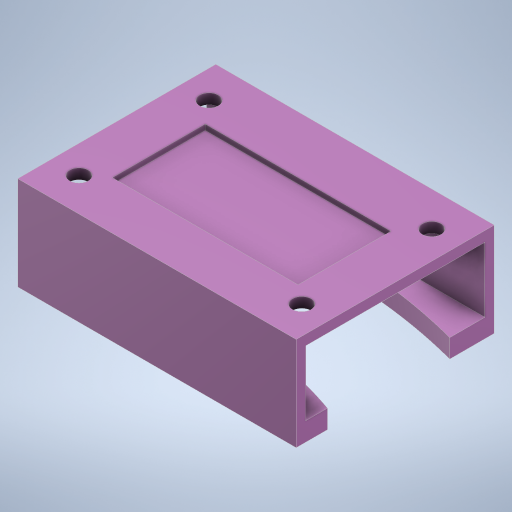
# Autodesk Inventor part: Battery Cage
Saved by Autodesk Inventor 2023 (Build 270158000, 158)
## iProperties
Created: 2022-10-27
Part Number: Battery Cage
Material: PLA Plastic
Document SubType Name: Modeling
Designer: cheng
Density: 1.25002 g/cm^3
Appearance: Generic
Mass: 171.099 g
Surface Area: 610.398 cm^2
Volume: 136.877 cm^3
Author: cheng
Autodesk Inventor part; units mm, degrees
ref_plane "YZ Plane" through (0, 0, 0) normal (1, 0, 0) x (0, 1, 0)
ref_plane "XZ Plane" through (0, 0, 0) normal (0, 1, 0) x (-1, 0, 0)
ref_plane "XY Plane" through (0, 0, 0) normal (0, 0, 1) x (1, 0, 0)
sketch "Sketch1" plane through (0, 0, 0) normal (0, 1, 0) x (-1, 0, 0)
  line L0 (75, -60) -> (-75, -60)
  line L1 (-75, -60) -> (-75, 60)
  line L2 (-75, 60) -> (75, 60)
  line L3 (75, 60) -> (75, -60)
  line L4 (75, -60) -> (-75, 60) construction
  line L5 (-75, -60) -> (75, 60) construction
  point P0 (0, 0)
  dimension "d0" = 120
  dimension "d1" = 150
  constraints: 12 end point, 2 midpoint, 2 parallel, 1 horizontal, 1 perpendicular
  measures "d0" distance of L2.end L0.start
  measures "d1" distance of L0.start L0.end
extrude "Extrusion1" add sketch "Sketch1" along normal blind 50.5
sketch "Sketch14" plane through (0, 0, 0) normal (0, 1, 0) x (1, 0, 0)
  line L0 (-75, -60) -> (75, -60) projected
  line L1 (75, -60) -> (75, 60) projected
  line L2 (75, 60) -> (-75, 60) projected
  line L3 (-75, 60) -> (-75, -60) projected
  line L4 (0, 0) -> (0, -250) construction
  circle A0 centre (0, -250) radius 260
  circle A1 centre (0, -250) radius 291.5
  circle A2 centre (0, -250) radius 228.5
  point P0 (75, 31.6864)
  point P1 (-75, 31.6864)
  point P2 (-75, -34.1592)
  point P3 (75, -34.1592)
  dimension "d52" = 250
  dimension "d53" = 520
  dimension "d54" = 583
  dimension "d55" = 457
  constraints: 4 coincident, 3 centre point, 2 end point, 1 vertical
  measures "d52" distance of L4.start L4.end
  measures "d53" diameter of A0
  measures "d54" diameter of A1
  measures "d55" diameter of A2
extrude "Extrusion13" cut sketch "Sketch14" along normal blind 45 contours L3 A0 L1 A2 | L3 A1 L1 A0 picked at (-61.8874, -8.4536) picked at (67.9829, 11.6585)
sketch "Sketch15" plane through (0, 45, 0) normal (0, -1, 0) x (1, 0, 0)
  line L0 (0, 0) -> (0, 250) construction
  circle A0 centre (0, 250) radius 260
  circle A1 centre (0, 250) radius 302.5
  circle A2 centre (0, 250) radius 217.5
  line L1 (-75, 60) -> (75, 60) projected
  line L2 (75, 60) -> (75, -60) projected
  line L3 (75, -60) -> (-75, -60) projected
  line L4 (-75, -60) -> (-75, 60) projected
  point P0 (-75, -43.055)
  point P1 (75, -43.055)
  point P2 (75, 45.8401)
  point P3 (-75, 45.8401)
  dimension "d58" = 250
  dimension "d59" = 520
  dimension "d60" = 605
  dimension "d61" = 435
  constraints: 4 coincident, 3 centre point, 2 end point, 1 vertical
  measures "d58" distance of L0.start L0.end
  measures "d59" diameter of A0
  measures "d60" diameter of A1
  measures "d61" diameter of A2
extrude "Extrusion14" cut sketch "Sketch15" along normal blind 35 contours L4 A2 L2 A0 | A0 L2 A1 L4 picked at (-61.9043, 12.2496) picked at (67.9829, -15.4481)
sketch "Sketch16" plane through (0, 50.5, 0) normal (0, 1, 0) x (1, 0, 0)
  line L0 (0, 0) -> (50, 0) construction
  line L1 (0, 0) -> (-50, 0) construction
  line L2 (-50, 0) -> (-50, -25)
  line L3 (-50, -25) -> (50, -25)
  line L4 (50, -25) -> (50, 0)
  line L5 (50, 0) -> (50, 25)
  line L6 (50, 25) -> (-50, 25)
  line L7 (-50, 25) -> (-50, 0)
  dimension "d64" = 50
  dimension "d65" = 50
  dimension "d66" = 25
  dimension "d67" = 25
  constraints: 16 end point, 4 perpendicular, 2 horizontal, 2 vertical
  measures "d64" distance of L0.start L0.end
  measures "d65" distance of L0.start L1.end
  measures "d66" distance of L1.end L2.end
  measures "d67" distance of L0.end L5.end
extrude "Extrusion15" cut sketch "Sketch16" against normal blind 3
sketch "Sketch17" plane through (0, 10, 0) normal (0, 1, 0) x (1, 0, 0)
  line L0 (0, 0) -> (-33, 0) construction
  line L1 (0, 0) -> (33, 0) construction
  line L2 (33, 0) -> (33, -35.018)
  arc A0 (75, -45.8401) -> (-75, -45.8401) centre (0, -250) ccw projected
  line L3 (33, 0) -> (68.018, 0) construction
  line L4 (-31.2481, 0) -> (6.0348, 0) construction
  line L5 (-33, 0) -> (-33, -35.018)
  line L6 (-33, 0) -> (2.018, 0) construction
  line L7 (-33, 0) -> (-33, 50.6946)
  arc A1 (75, 43.055) -> (-75, 43.055) centre (0, -250) ccw projected
  line L8 (-33, 0) -> (17.6946, 0) construction
  line L9 (33, 0) -> (33, 50.6946)
  line L10 (33, 0) -> (83.6946, 0) construction
  dimension "d70" = 33
  dimension "d71" = 33
  dimension "d72" = 90
  dimension "d74" = 90
  dimension "d75" = 90
  dimension "d76" = 90
  constraints: 22 end point, 7 horizontal, 4 perpendicular, 4 point on circle, 1 point on line
  measures "d70" distance of L0.start L0.end
  measures "d71" distance of L0.start L1.end
  measures "d72" angle of L2 L3
  measures "d74" angle of L5 L6
  measures "d75" angle of L8 L7
  measures "d76" angle of L10 L9
extrude "Extrusion16" cut sketch "Sketch17" against normal blind 7
sketch "Sketch18" plane through (75, 0, -60) normal (1, 0, 0) x (0, 0, -1)
  line L0 (-94.1592, 10) -> (-105.8401, 10) projected
  line L1 (-105.8401, 10) -> (-105.8401, 45) projected
  line L2 (-105.8401, 45) -> (-16.945, 45) projected
  line L3 (-16.945, 45) -> (-16.945, 10) projected
  line L4 (-16.945, 10) -> (-28.3136, 10) projected
  line L5 (-28.3136, 10) -> (-28.3136, 0) projected
  line L6 (-28.3136, 0) -> (0, 0) projected
  line L7 (0, 0) -> (0, 50.5) projected
  line L8 (-120, 50.5) -> (0, 50.5) projected
  line L9 (-120, 0) -> (-120, 50.5) projected
  line L10 (-120, 0) -> (-94.1592, 0) projected
  line L11 (-94.1592, 0) -> (-94.1592, 10) projected
  line L12 (-60, 0) -> (-60, 50.5) construction
  line L13 (-94.1592, 10) -> (-28.3136, 10)
  line L14 (-60, 10) -> (-111, 10)
  line L15 (-111, 10) -> (-111, 45)
  line L16 (-16.945, 10) -> (-9.3054, 10) projected
  line L17 (-28.3136, 10) -> (-9.3054, 10)
  line L18 (-9.3054, 10) -> (-9.3054, 3) projected
  line L19 (-9.3054, 10) -> (-9.3054, 45)
  line L20 (-111, 45) -> (-105.8401, 45)
  line L21 (-9.3054, 45) -> (-16.945, 45)
  line L22 (-111, 45) -> (-116, 45)
  line L23 (-116, 45) -> (-116, 10)
  line L24 (-116, 10) -> (-111, 10)
  line L25 (-9.3054, 45) -> (-4.3054, 45)
  line L26 (-4.3054, 45) -> (-4.3054, 10)
  line L27 (-4.3054, 10) -> (-9.3054, 10)
  line L28 (-116, 45) -> (-116, 50.5)
  line L29 (-116, 10) -> (-116, 0)
  line L30 (-94.1592, 0) -> (-120, 0) projected
  line L31 (-4.3054, 45) -> (-4.3054, 50.5)
  line L32 (-4.3054, 10) -> (-4.3054, 0)
  line L33 (-111, 45) -> (-111, 50.5)
  line L34 (-9.3054, 45) -> (-9.3054, 50.5)
  line L35 (-9.3054, 10) -> (-9.3054, 0)
  line L36 (-111, 10) -> (-111, 0)
  point P0 (-9.3054, 3)
  dimension "d79" = 51
  dimension "d81" = 5
  dimension "d82" = 5
  constraints: 44 end point, 17 point on line, 8 perpendicular, 3 collinear, 2 horizontal, 2 vertical, 1 midpoint
  measures "d79" distance of L14.start L14.end
  measures "d81" distance of L15.end L22.end
  measures "d82" distance of L19.end L25.end
extrude "Extrusion17" cut sketch "Sketch18" against normal up to surface (150 mm away) contours L0 L1 L2 L3 L4 L13 | L24 L23 L22 L15 | L36 L10 L29 L24 | L21 L19 L16 L3 | L22 L28 L8 L33 | L29 L10 L9 L8 L28 L23 | L31 L8 L7 L6 L32 L26
sketch "Sketch19" plane through (0, 50.5, 0) normal (0, 1, 0) x (1, 0, 0)
  line L0 (75, 55.6946) -> (-75, 55.6946) projected
  line L1 (-75, 55.6946) -> (-75, -51) projected
  line L2 (-75, -51) -> (75, -51) projected
  line L3 (75, -51) -> (75, 55.6946) projected
  line L4 (50, 25) -> (50, -25) projected
  line L5 (50, -25) -> (-50, -25) projected
  line L6 (-50, -25) -> (-50, 25) projected
  line L7 (-50, 25) -> (50, 25) projected
  line L8 (50, 25) -> (50, -25) construction
  line L9 (50, -25) -> (-50, 25) construction
  line L10 (-50, -25) -> (-50, 25) construction
  line L11 (50, 25) -> (-50, -25) construction
  line L12 (50, -25) -> (-50, -25) construction
  line L13 (50, -25) -> (50, -33) construction
  line L14 (50, -33) -> (60, -33) construction
  line L15 (50, 25) -> (50, 37) construction
  line L16 (50, 37) -> (60, 37) construction
  circle A0 centre (60, -33) radius 5
  circle A1 centre (60, 37) radius 5
  line L17 (0, -51) -> (0, 55.6946) construction
  circle A2 centre (-60, -33) radius 5
  circle A3 centre (-60, 37) radius 5
  dimension "d93" = 8
  dimension "d94" = 10
  dimension "d95" = 12
  dimension "d96" = 10
  dimension "d97" = 90
  dimension "d98" = 10
  dimension "d99" = 10
  constraints: 14 end point, 4 centre point, 2 coincident, 2 midpoint, 2 perpendicular, 2 symmetric about line, 2 vertical, 2 other
  measures "d93" distance of L4.end L13.end
  measures "d94" distance of L13.end L14.end
  measures "d95" distance of L4.start L15.end
  measures "d96" distance of L15.end L16.end
  measures "d97" angle of L15 L16
  measures "d98" diameter of A0
  measures "d99" diameter of A1
extrude "Extrusion18" cut sketch "Sketch19" against normal blind 10 contours A0 | A1 | A2 | A3
body "Solid1"
